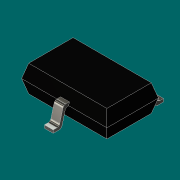
# Autodesk Inventor part: SOT23-3
Saved by Autodesk Inventor 2016 (Build 200138000, 138)
## iProperties
Created: 2015-10-16
Part Number: SOT23-3
Material: ABS Plastic
Document SubType Name: Modeling
Designer: Sawaiz
Density: 1.06 g/cm^3
Appearance: Smooth - Black
Author: Sawaiz
Autodesk Inventor part; units mm, degrees
ref_plane "XZ Plane" through (0, 0, 0) normal (0, 1, 0) x (-1, 0, 0)
ref_plane "XY Plane" through (0, 0, 0) normal (0, 0, 1) x (1, 0, 0)
sketch "Sketch1" plane through (0, 0, 0) normal (0, 0, 1) x (1, 0, 0)
  line L0 (0.875, -1.45) -> (-0.875, -1.45)
  line L1 (-0.875, -1.45) -> (-0.875, 1.45)
  line L2 (-0.875, 1.45) -> (0.875, 1.45)
  line L3 (0.875, 1.45) -> (0.875, -1.45)
  line L4 (0.875, -1.45) -> (-0.875, 1.45) construction
  line L5 (-0.875, -1.45) -> (0.875, 1.45) construction
  point P0 (0, 0)
  dimension "d0" = 1.75
  dimension "d1" = 2.9
  constraints: 12 end point, 2 midpoint, 2 parallel, 1 horizontal, 1 perpendicular
  measures "d0" distance of L1.end L2.end
  measures "d1" distance of L0.end L1.end
extrude "Extrusion1" add sketch "Sketch1" along normal blind 0.9
sketch "Sketch2" plane through (-0.875, 1.45, 0) normal (0, 1, 0) x (1, 0, 0)
  line L0 (0, 0) -> (1.75, 0) projected
  line L1 (0, 0) -> (0, -0.9) projected
  line L2 (1.75, -0.9) -> (0, -0.9) projected
  line L3 (1.75, 0) -> (1.75, -0.9) projected
  line L4 (1.75, -0.45) -> (1.6294, -0.9)
  line L5 (0, -0.9) -> (1.75, -0.9) projected
  line L6 (1.75, -0.45) -> (1.6294, 0)
  line L7 (1.75, 0) -> (0, 0) projected
  line L8 (0.1206, 0) -> (0, -0.45)
  line L9 (0.1206, -0.9) -> (0, -0.45)
  point P0 (0.875, 0)
  dimension "d4" = 15
  dimension "d5" = 15
  constraints: 8 end point, 4 point on line, 2 equal length, 2 midpoint
  measures "d4" angle of L3 L4
  measures "d5" angle of L3 L6
extrude "Extrusion2" cut sketch "Sketch2" against normal through all contours L0 L6 L4 L2 L9 L8 keep common part
ref_plane "Work Plane1" through (1.25, 0, 0) normal (1, 0, 0) x (0, 1, 0)
sketch "Sketch4" plane through (1.25, 0, 0) normal (1, 0, 0) x (0, 1, 0)
  line L0 (1.45, 0.9) -> (-1.45, 0.9) projected
  line L1 (-1.45, 0) -> (1.45, 0) projected
  line L2 (-1.3294, 0) -> (-1.45, 0.45)
  line L3 (-1.45, 0.45) -> (-1.3294, 0.9)
  line L4 (1.3294, 0.9) -> (1.45, 0.45)
  line L5 (1.45, 0.45) -> (1.3294, 0)
  line L6 (1.45, 0) -> (1.45, 0.45) projected
  line L7 (-1.45, 0.45) -> (-1.45, 0) projected
  point P0 (0, 0)
  dimension "d10" = 15
  dimension "d11" = 15
  dimension "d12" = 0
  constraints: 8 end point, 4 point on line, 3 equal length
  measures "d10" angle of L6 L5
  measures "d11" angle of L7 L2
  measures "d12" distance from line of L7 L2.end
extrude "Extrusion3" cut sketch "Sketch4" against normal through all contours L4 L5 L1 L2 L3 L0 keep common part
sketch "Sketch5" plane through (0, 0, 0) normal (0, 1, 0) x (-1, 0, 0)
  line L0 (-0.875, 0.45) -> (-0.7544, 0.9) projected
  line L1 (-0.7544, 0) -> (-0.875, 0.45) projected
  line L2 (-0.875, 0.45) -> (-0.9733, 0.45)
  line L3 (-0.9733, 0.45) -> (-1.1206, -0.1)
  line L4 (-1.1206, -0.1) -> (-1.4, -0.1)
  line L5 (-1.4, -0.1) -> (-1.4, 0)
  line L6 (-1.4, 0) -> (-1.1974, 0)
  line L7 (-1.1974, 0) -> (-1.05, 0.55)
  line L8 (-1.05, 0.55) -> (-0.8482, 0.55)
  line L9 (0.7544, 0) -> (-0.7544, 0) projected
  point P0 (0, 0)
  point P1 (0, 0)
  dimension "d15" = 0.1
  dimension "d17" = 0.1
  dimension "d18" = 0.1
  dimension "d19" = 0.1
  dimension "d20" = 105
  dimension "d21" = 1.4
  dimension "d22" = 0.35
  constraints: 14 end point, 3 parallel, 2 perpendicular, 1 coincident, 1 horizontal, 1 point on line
  measures "d15" distance between parallel lines of L4 L6
  measures "d17" distance between parallel lines of L8 L2
  measures "d18" distance between parallel lines of L7 L3
  measures "d19" distance between parallel lines of L4 L9
  measures "d20" angle of L3 L2
  measures "d21" distance from line of L5 point (0, 0)
  measures "d22" distance from line of L5 L7.end
extrude "Extrusion4" add sketch "Sketch5" along normal mid plane 0.3 separate body
fillet "Fillet1" radius 0.1 4 edges at (1.1974, 0, 0) (1.05, 0, 0.55) (1.1206, 0, -0.1) (0.9733, 0, 0.45)
pattern_linear "Rectangular Pattern1" count 3 spacing 0.95 along (0, 1, 0) of "Extrusion4", "Fillet1" first direction both ways yes bodies 2
mirror "Mirror1" about plane through (0, 0, 0) normal (1, 0, 0) of "Extrusion4", "Rectangular Pattern1" bodies 2
sketch "Sketch7" plane through (-1.4, 0.15, -0.1) normal (0, 1, 0) x (1, 0, 0)
  line L0 (0.5518, -0.65) -> (0.525, -0.55) projected
  line L1 (0.35, -0.65) -> (0.5518, -0.65) projected
  line L2 (0.2026, -0.1) -> (0.35, -0.65) projected
  line L3 (0, -0.1) -> (0.2026, -0.1) projected
  line L4 (0, 0) -> (0, -0.1) projected
  line L5 (0.2794, 0) -> (0, 0) projected
  line L6 (0.4267, -0.55) -> (0.2794, 0) projected
  line L7 (0.525, -0.55) -> (0.4267, -0.55) projected
  arc A0 (0.2992, -0.0741) -> (0.2026, 0) centre (0.2026, -0.1) ccw projected
  line L8 (0, 0) -> (0.2026, 0) projected
  line L9 (0, -0.1) -> (0, 0) projected
  line L10 (0.1259, -0.1) -> (0, -0.1) projected
  arc A1 (0.2225, -0.1741) -> (0.1259, -0.1) centre (0.1259, -0.2) ccw projected
  line L11 (0.3301, -0.5759) -> (0.2225, -0.1741) projected
  arc A2 (0.3301, -0.5759) -> (0.4267, -0.65) centre (0.4267, -0.55) ccw projected
  line L12 (0.5518, -0.65) -> (0.4267, -0.65) projected
  line L13 (0.525, -0.55) -> (0.5518, -0.65) projected
  line L14 (0.5035, -0.55) -> (0.525, -0.55) projected
  arc A3 (0.4069, -0.4759) -> (0.5035, -0.55) centre (0.5035, -0.45) ccw projected
  line L15 (0.2992, -0.0741) -> (0.4069, -0.4759) projected
  point P0 (1.4, -0.1)
extrude "Extrusion6" cut sketch "Sketch7" against normal up to surface (0.3 mm away) bodies 2
sketch "Sketch8" plane through (1.1974, -1.1, -0.1) normal (0, -1, 0) x (1, 0, 0)
  arc A0 (-0.0966, 0.0741) -> (0, 0) centre (0, 0.1) ccw projected
  line L0 (0, 0) -> (0.2026, 0) projected
  line L1 (0.2026, 0) -> (0.2026, 0.1) projected
  line L2 (0.2026, 0.1) -> (0.0767, 0.1) projected
  arc A1 (-0.0199, 0.1741) -> (0.0767, 0.1) centre (0.0767, 0.2) ccw projected
  line L3 (-0.0199, 0.1741) -> (-0.1275, 0.5759) projected
  arc A2 (-0.1275, 0.5759) -> (-0.2241, 0.65) centre (-0.2241, 0.55) ccw projected
  line L4 (-0.2241, 0.65) -> (-0.3492, 0.65) projected
  line L5 (-0.3492, 0.65) -> (-0.3224, 0.55) projected
  line L6 (-0.3224, 0.55) -> (-0.3008, 0.55) projected
  arc A3 (-0.2042, 0.4759) -> (-0.3008, 0.55) centre (-0.3008, 0.45) ccw projected
  line L7 (-0.2042, 0.4759) -> (-0.0966, 0.0741) projected
  point P0 (-1.1974, 0.1)
extrude "Extrusion7" cut sketch "Sketch8" against normal up to surface (0.3 mm away) bodies 2
sketch "Sketch9" plane through (1.1974, 1.1, -0.1) normal (0, 1, 0) x (1, 0, 0)
  arc A0 (0, 0) -> (-0.0966, -0.0741) centre (0, -0.1) ccw projected
  line L0 (-0.0966, -0.0741) -> (-0.2042, -0.4759) projected
  arc A1 (-0.3008, -0.55) -> (-0.2042, -0.4759) centre (-0.3008, -0.45) ccw projected
  line L1 (-0.3008, -0.55) -> (-0.3224, -0.55) projected
  line L2 (-0.3224, -0.55) -> (-0.3492, -0.65) projected
  line L3 (-0.3492, -0.65) -> (-0.2241, -0.65) projected
  arc A2 (-0.2241, -0.65) -> (-0.1275, -0.5759) centre (-0.2241, -0.55) ccw projected
  line L4 (-0.1275, -0.5759) -> (-0.0199, -0.1741) projected
  arc A3 (0.0767, -0.1) -> (-0.0199, -0.1741) centre (0.0767, -0.2) ccw projected
  line L5 (0.0767, -0.1) -> (0.2026, -0.1) projected
  line L6 (0.2026, -0.1) -> (0.2026, 0) projected
  line L7 (0.2026, 0) -> (0, 0) projected
  point P0 (-1.1974, -0.1)
extrude "Extrusion8" cut sketch "Sketch9" against normal up to surface (0.3 mm away) bodies 2
body "Solid1"
body "Solid2"
